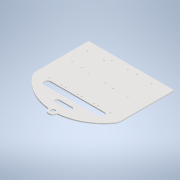
# Autodesk Inventor part: Top Plate
Saved by Autodesk Inventor 2020 (Build 240168000, 168)
## iProperties
Created: 2020-02-08
Part Number: Top Plate
Material: Generic
Document SubType Name: Modeling
Designer: holtat
Density: 1 g/cm^3
Appearance: Default
Author: holtat
Autodesk Inventor part; units mm, degrees
ref_plane "YZ Plane" through (0, 0, 0) normal (1, 0, 0) x (0, 1, 0)
ref_plane "XZ Plane" through (0, 0, 0) normal (0, 1, 0) x (-1, 0, 0)
ref_plane "XY Plane" through (0, 0, 0) normal (0, 0, 1) x (1, 0, 0)
sketch "Sketch1" plane through (0, 0, 0) normal (0, 1, 0) x (-1, 0, 0)
  line L0 (127, -82.55) -> (-127, -82.55)
  line L1 (-127, -82.55) -> (-127, 82.55)
  line L2 (127, 82.55) -> (127, -82.55)
  circle A0 centre (0, 150.7034) radius 6.35
  arc A1 (12.7, 150.7034) -> (-12.7, 150.7034) centre (0, 150.7034) ccw
  line L3 (79.375, 87.2034) -> (-79.375, 87.2034) construction
  line L4 (79.375, 96.7284) -> (-79.375, 96.7284)
  line L5 (-79.375, 77.6784) -> (79.375, 77.6784)
  arc A2 (79.375, 77.6784) -> (79.375, 96.7284) centre (79.375, 87.2034) ccw
  arc A3 (-79.375, 96.7284) -> (-79.375, 77.6784) centre (-79.375, 87.2034) ccw
  line L6 (94.1705, 96.449) -> (49.3141, 96.449) projected
  circle A4 centre (80.3783, 87.2034) radius 3.175 projected
  circle A5 centre (63.1063, 87.2034) radius 3.175 projected
  circle A6 centre (32.3469, 87.2034) radius 3.175 projected
  circle A7 centre (15.0749, 87.2034) radius 3.175 projected
  circle A8 centre (-15.6845, 87.2034) radius 3.175 projected
  circle A9 centre (-32.9565, 87.2034) radius 3.175 projected
  circle A10 centre (-63.7159, 87.2034) radius 3.175 projected
  circle A11 centre (-80.9879, 87.2034) radius 3.175 projected
  arc A12 (127, 82.55) -> (12.7, 150.7034) centre (0, -0.5186) ccw
  arc A13 (-12.7, 150.7034) -> (-127, 82.55) centre (0, -0.5186) ccw
  point P0 (0, 0)
  point P1 (127, 0)
  point P2 (0, -82.55)
  point P3 (0, 87.2034)
  point P4 (0, 87.2034)
  dimension "d0" = 12.7
  dimension "d1" = 6.35
  dimension "d4" = 254
  dimension "d5" = 19.05
  dimension "d6" = 177.8
  dimension "d10" = 63.5
  dimension "d15" = 165.1
  constraints: 14 end point, 10 point on circle, 6 centre point, 4 horizontal alignment, 4 tangent, 3 coincident, 3 midpoint, 3 parallel, 3 vertical alignment, 2 horizontal, 1 concentric, 1 perpendicular
  measures "d0" diameter of A0
  measures "d1" radial gap between concentric circles of A1 A0
  measures "d4" distance of L0.start L0.end
  measures "d5" distance between parallel lines of L4 L5
  measures "d10" distance from line of L3 A0.centre
  measures "d15" distance of L2.start L0.start
extrude "Extrusion1" add sketch "Sketch1" along normal mid plane 3.175 contours L0 L1 A13 A1 A12 L2
sketch "Sketch2" plane through (0, 1.5875, 0) normal (0, 1, 0) x (1, 0, 0)
  line L0 (-49.3141, -31.933) -> (-94.1705, -31.933)
  line L1 (-94.1705, -31.933) -> (-94.1705, -96.449)
  line L2 (-94.1705, -96.449) -> (-49.3141, -96.449)
  line L3 (-49.3141, -96.449) -> (-49.3141, -31.933)
  circle A0 centre (-53.5813, -71.049) radius 1.5875
  circle A1 centre (-89.9033, -71.049) radius 1.5875
  line L4 (-1.2827, -31.933) -> (-46.1391, -31.933)
  line L5 (-46.1391, -31.933) -> (-46.1391, -96.449)
  line L6 (-46.1391, -96.449) -> (-1.2827, -96.449)
  line L7 (-1.2827, -96.449) -> (-1.2827, -31.933)
  circle A2 centre (-5.5499, -71.049) radius 1.5875
  circle A3 centre (-41.8719, -71.049) radius 1.5875
  line L8 (46.7487, -31.933) -> (1.8923, -31.933)
  line L9 (1.8923, -31.933) -> (1.8923, -96.449)
  line L10 (1.8923, -96.449) -> (46.7487, -96.449)
  line L11 (46.7487, -96.449) -> (46.7487, -31.933)
  circle A4 centre (42.4815, -71.049) radius 1.5875
  circle A5 centre (6.1595, -71.049) radius 1.5875
  line L12 (94.7801, -31.933) -> (49.9237, -31.933)
  line L13 (49.9237, -31.933) -> (49.9237, -96.449)
  line L14 (49.9237, -96.449) -> (94.7801, -96.449)
  line L15 (94.7801, -96.449) -> (94.7801, -31.933)
  circle A6 centre (90.5129, -71.049) radius 1.5875
  circle A7 centre (54.1909, -71.049) radius 1.5875
  circle A8 centre (-68.834, 3.81) radius 1.5875
  circle A9 centre (-54.6269, 54.61) radius 1.5875
  circle A10 centre (-97.79, 3.81) radius 1.5875
  circle A11 centre (-102.87, 54.61) radius 1.5875
  line L16 (-61.3664, 81.9424) -> (-73.3552, 81.9424)
  line L17 (-73.3552, 81.9424) -> (-73.3552, 69.85)
  line L18 (-73.3552, 69.85) -> (-105.41, 69.85)
  line L19 (-105.41, 69.85) -> (-105.41, 1.27)
  line L20 (-105.41, 1.27) -> (-52.324, 1.27)
  line L21 (-52.324, 1.27) -> (-52.324, 69.85)
  line L22 (-52.324, 69.85) -> (-61.3664, 69.85)
  line L23 (-61.3664, 69.85) -> (-61.3664, 81.9424)
  line L24 (9.144, -5.08) -> (9.144, 69.85)
  line L25 (9.144, 69.85) -> (-45.974, 69.85)
  line L26 (-45.974, 69.85) -> (-45.974, -5.08)
  line L27 (-45.974, -5.08) -> (9.144, -5.08)
  circle A12 centre (-42.418, -1.524) radius 1.4605
  circle A13 centre (5.588, -1.524) radius 1.4605
  circle A14 centre (5.588, 66.294) radius 1.4605
  circle A15 centre (-42.418, 66.294) radius 1.4605
  line L28 (78.994, -6.985) -> (78.994, 69.85)
  line L29 (78.994, 69.85) -> (28.194, 69.85)
  line L30 (28.194, 69.85) -> (28.194, -6.985)
  line L31 (28.194, -6.985) -> (78.994, -6.985)
  circle A16 centre (75.819, -3.81) radius 1.5875
  circle A17 centre (75.819, 66.675) radius 1.5875
  circle A18 centre (31.369, 66.675) radius 1.5875
  circle A19 centre (31.369, -3.81) radius 1.5875
  circle A20 centre (-102.87, 54.61) radius 1.5875
  circle A21 centre (-54.6269, 54.61) radius 1.5875
  circle A22 centre (-68.834, 3.81) radius 1.5875
  circle A23 centre (-97.79, 3.81) radius 1.5875
  circle A24 centre (-42.418, 66.294) radius 1.5875
  circle A25 centre (-42.418, -1.524) radius 1.5875
  circle A26 centre (5.588, -1.524) radius 1.5875
  circle A27 centre (5.588, 66.294) radius 1.5875
  circle A28 centre (31.369, 66.675) radius 1.5875
  circle A29 centre (75.819, 66.675) radius 1.5875
  circle A30 centre (75.819, -3.81) radius 1.5875
  circle A31 centre (31.369, -3.81) radius 1.5875
  circle A32 centre (90.5129, -71.049) radius 1.5875
  circle A33 centre (54.1909, -71.049) radius 1.5875
  circle A34 centre (42.4815, -71.049) radius 1.5875
  circle A35 centre (6.1595, -71.049) radius 1.5875
  circle A36 centre (-5.5499, -71.049) radius 1.5875
  circle A37 centre (-41.8719, -71.049) radius 1.5875
  circle A38 centre (-53.5813, -71.049) radius 1.5875
  circle A39 centre (-89.9033, -71.049) radius 1.5875
  point P0 (0, 0)
extrude "Extrusion2" cut sketch "Sketch2" against normal through all contours A0 | A1 | A2 | A3 | A4 | A5 | A6 | A7 | A8 | A9 | A10 | A11 | A12 | A13 | A14 | A15 | A16 | A17 | A18 | A19 | A24 | A27
fillet "Fillet1" radius 25.4 2 edges at (127, 0, 82.55) (-127, 0, 82.55)
sketch "Sketch3" plane through (0, 1.5875, 0) normal (0, 1, 0) x (1, 0, 0)
  arc A0 (-127, -74.6004) -> (-122.0238, -89.701) centre (-101.6, -74.6004) ccw projected
  arc A1 (-122.0238, -89.701) -> (-12.7, -150.7034) centre (0, 0.5186) ccw projected
  arc A2 (-12.7, -150.7034) -> (12.7, -150.7034) centre (0, -150.7034) ccw projected
  arc A3 (12.7, -150.7034) -> (122.0238, -89.701) centre (0, 0.5186) ccw projected
  arc A4 (122.0238, -89.701) -> (127, -74.6004) centre (101.6, -74.6004) ccw projected
  line L0 (127, -74.6004) -> (127, 82.55) projected
  line L1 (127, 82.55) -> (-127, 82.55) projected
  line L2 (-127, 82.55) -> (-127, -74.6004) projected
  circle A5 centre (-53.5813, -71.049) radius 1.5875 projected
  circle A6 centre (54.1909, -71.049) radius 1.5875 projected
  circle A7 centre (31.369, 66.675) radius 1.5875 projected
  circle A8 centre (-42.418, -1.524) radius 1.4605 projected
  circle A9 centre (-97.79, 3.81) radius 1.5875 projected
  circle A10 centre (-68.834, 3.81) radius 1.5875 projected
  circle A11 centre (5.588, -1.524) radius 1.4605 projected
  circle A12 centre (31.369, -3.81) radius 1.5875 projected
  circle A13 centre (42.4815, -71.049) radius 1.5875 projected
  circle A14 centre (-5.5499, -71.049) radius 1.5875 projected
  circle A15 centre (-89.9033, -71.049) radius 1.5875 projected
  circle A16 centre (90.5129, -71.049) radius 1.5875 projected
  circle A17 centre (75.819, 66.675) radius 1.5875 projected
  circle A18 centre (-42.418, 66.294) radius 1.5875 projected
  circle A19 centre (-102.87, 54.61) radius 1.5875 projected
  circle A20 centre (-54.6269, 54.61) radius 1.5875 projected
  circle A21 centre (5.588, 66.294) radius 1.5875 projected
  circle A22 centre (75.819, -3.81) radius 1.5875 projected
  circle A23 centre (6.1595, -71.049) radius 1.5875 projected
  circle A24 centre (-41.8719, -71.049) radius 1.5875 projected
  line L3 (79.375, -96.7284) -> (-79.375, -96.7284) projected
  arc A25 (-79.375, -77.6784) -> (-79.375, -96.7284) centre (-79.375, -87.2034) ccw projected
  line L4 (-79.375, -77.6784) -> (79.375, -77.6784) projected
  arc A26 (79.375, -96.7284) -> (79.375, -77.6784) centre (79.375, -87.2034) ccw projected
  circle A27 centre (0, -150.7034) radius 6.35 projected
  line L5 (-25.4, -118.9534) -> (25.4, -118.9534) construction
  line L6 (-19.05, -125.3034) -> (19.05, -125.3034)
  line L7 (19.05, -112.6034) -> (-19.05, -112.6034)
  arc A28 (-19.05, -112.6034) -> (-19.05, -125.3034) centre (-19.05, -118.9534) ccw
  arc A29 (19.05, -125.3034) -> (19.05, -112.6034) centre (19.05, -118.9534) ccw
  point P0 (0, 0)
  point P1 (0, -118.9534)
  dimension "d17" = 50.8
  dimension "d18" = 12.7
  dimension "d19" = 25.4
  constraints: 8 end point, 6 point on circle, 4 tangent, 2 centre point, 2 point on line, 1 horizontal, 1 midpoint, 1 parallel, 1 vertical alignment
  measures "d17" distance of L5.start L5.end
  measures "d18" distance between parallel lines of L7 L6
  measures "d19" distance from line of A2.centre L6
extrude "Extrusion3" cut sketch "Sketch3" against normal blind 3.175 contours A28 L7 A29 L6
body "Solid1"
